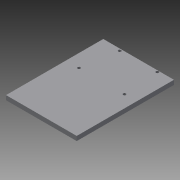
# Autodesk Inventor part: sensor bottom
Saved by Autodesk Inventor 2015 (Build 190159000, 159)
## iProperties
Created: 2014-11-13
Part Number: sensor bottom
Material: Generic
Document SubType Name: Modeling
Designer: ericd_000
Density: 1 g/cm^3
Appearance: Default
Author: ericd_000
Autodesk Inventor part; units mm, degrees
ref_plane "YZ Plane" through (0, 0, 0) normal (1, 0, 0) x (0, 1, 0)
ref_plane "XZ Plane" through (0, 0, 0) normal (0, 1, 0) x (-1, 0, 0)
ref_plane "XY Plane" through (0, 0, 0) normal (0, 0, 1) x (1, 0, 0)
sketch "Sketch1" plane through (0, 0, 0) normal (0, 0, 1) x (1, 0, 0)
  line L0 (-80, 110) -> (80, 110)
  line L1 (80, 110) -> (80, -110)
  line L2 (80, -110) -> (-80, -110)
  line L3 (-80, -110) -> (-80, 110)
  point P0 (0, 0)
  point P1 (-80, 0)
  point P2 (0, 110)
  dimension "d0" = 160
  dimension "d1" = 220
  constraints: 8 end point, 2 midpoint, 2 parallel, 1 horizontal, 1 horizontal alignment, 1 perpendicular, 1 vertical alignment
  measures "d0" distance of L0.start L0.end
  measures "d1" distance of L2.end L0.start
extrude "Extrusion1" add sketch "Sketch1" along normal blind 10
sketch "Sketch2" plane through (0, 0, 10) normal (0, 0, 1) x (1, 0, 0)
  circle A0 centre (52.3704, 25.8177) radius 1.7
  circle A1 centre (52.3704, 25.8177) radius 3.15
  circle A2 centre (-50.6296, 25.8177) radius 1.7
  circle A3 centre (-50.6296, 25.8177) radius 3.15
  circle A4 centre (-38.1296, 105.3177) radius 3.15
  circle A5 centre (46.0364, 106.2745) radius 1.7
  circle A6 centre (46.0364, 106.2745) radius 3.15
  circle A7 centre (52.3704, 25.8177) radius 3.15
  circle A8 centre (-50.6296, 25.8177) radius 3.15
  circle A9 centre (-38.1296, 105.3177) radius 3.15
  circle A10 centre (46.0364, 106.2745) radius 3.15
  point P0 (0, 0)
  point P1 (8.7862, 59.2077)
  constraints: 11 centre point, 5 concentric, 3 coincident
extrude "Extrusion2" cut sketch "Sketch2" against normal up to surface (10 mm away) contours A0 | A1 | A2 | A3 | A4 | A5 | A6
body "Solid1"
